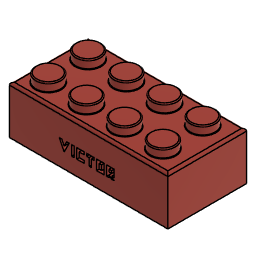
Week 2_Task 1_Ohene (Autodesk Fusion 360 design; units mm, degrees)
Autodesk Fusion 360 part; units mm, degrees
sketch "Sketch1" plane through (0, 0, 0) normal (0, 0, 1) x (1, 0, 0) in component "2x8 Block"
  line L0 (0, 0) -> (31.8, 0)
  line L1 (31.8, 0) -> (31.8, 15.8)
  line L2 (31.8, 15.8) -> (0, 15.8)
  line L3 (0, 15.8) -> (0, 0)
  dimension "d1" = 31.8
  dimension "d2" = 15.8
  constraint horizontal L0
  constraint vertical L1
  constraint horizontal L2
  constraint vertical L3
  constraint coincident L0.start L3.end
  measures "d1" distance of L0.start L0.end
  measures "d2" distance of L0.start L2.end
extrude "Extrude1" add sketch "Sketch1" along normal blind 9.6 in component "2x8 Block"
sketch "Sketch2" plane through (0, 0, 9.6) normal (0, 0, 1) x (-1, 0, 0) in component "2x8 Block"
  line L0 (0, -15.8) -> (0, 0)
  line L1 (0, 0) -> (-31.8, 0)
  line L2 (-31.8, 0) -> (-31.8, -15.8)
  line L3 (-31.8, -15.8) -> (0, -15.8)
  circle A0 centre (-3.9, -11.9) radius 2.5
  dimension "d5" = 5
  dimension "d6" = 3.9
  dimension "d7" = 3.9
  measures "d5" diameter of A0
  measures "d6" distance of L3 A0.centre
  measures "d7" distance of L0 A0.centre
extrude "Extrude2" add sketch "Sketch2" along normal blind 1.7 contours A0 in component "2x8 Block"
pattern_linear "R-Pattern1" count 2 spacing 8 along (0, -1, 0) count 4 spacing 7.6667 along (1, 0, 0) of "Extrude2" in component "2x8 Block"
shell "Shell1" thickness 1.49 removed faces 1 at (21.2, 5.2667, 0) in component "2x8 Block"
sketch "Sketch3" plane through (0, 0, 8.11) normal (0, 0, -1) x (1, 0, 0) in component "2x8 Block"
  circle A0 centre (26.9, -3.9) radius 1.01
  circle A1 centre (26.9, -11.9) radius 1.01
  circle A2 centre (19.2333, -3.9) radius 1.01
  circle A3 centre (19.2333, -11.9) radius 1.01
  circle A4 centre (11.5667, -3.9) radius 1.01
  circle A5 centre (11.5667, -11.9) radius 1.01
  circle A6 centre (3.9, -3.9) radius 1.01
  circle A7 centre (3.9, -11.9) radius 1.01
  line L0 (1.49, -1.49) -> (1.49, -14.31)
  line L1 (1.49, -14.31) -> (30.31, -14.31)
  line L2 (30.31, -14.31) -> (30.31, -1.49)
  line L3 (30.31, -1.49) -> (1.49, -1.49)
  line L4 (11.5667, -3.9) -> (3.9, -11.9) construction
  circle A8 centre (7.7333, -7.9) radius 3.15
  circle A9 centre (7.7333, -7.9) radius 2.15
  dimension "d15" = 6.3
  dimension "d16" = -1
  constraint coincident A4.centre L4.start
  constraint coincident A7.centre L4.end
  constraint midpoint L4 A8.centre
  measures "d15" diameter of A8
extrude "Extrude3" add sketch "Sketch3" along normal blind 8.1 contours A8 in component "2x8 Block"
pattern_linear "R-Pattern2" count 3 spacing 8 along (1, 0, 0) of "Extrude3" in component "2x8 Block"
fillet "Fillet1" radius 0.2 8 edges at (6.2308, 12.804, 11.3) (6.2308, 4.804, 11.3) (13.8975, 4.804, 11.3) (13.8975, 12.804, 11.3) (21.5642, 12.804, 11.3) (21.5642, 4.804, 11.3) (29.2308, 4.804, 11.3) (29.2308, 12.804, 11.3) in component "2x8 Block"
fillet "Fillet2" radius 0.1 8 edges at (6.2308, 10.996, 9.6) (13.8975, 10.996, 9.6) (6.2308, 2.996, 9.6) (13.8975, 2.996, 9.6) (21.5642, 2.996, 9.6) (21.5642, 10.996, 9.6) (29.2308, 10.996, 9.6) (29.2308, 2.996, 9.6) in component "2x8 Block"
fillet "Fillet3" radius 0.5 4 edges at (0, 7.9, 9.6) (15.9, 15.8, 9.6) (15.9, 0, 9.6) (31.8, 7.9, 9.6) in component "2x8 Block"
sketch "Sketch4" plane through (0, 0, 0) normal (0, -1, 0) x (1, 0, 0) in component "2x8 Block"
  line L0 (31.8, 9.1) -> (0, 9.1)
  line L1 (0, 9.1) -> (0, 0)
  line L2 (0, 0) -> (31.8, 0)
  line L3 (31.8, 0) -> (31.8, 9.1)
  line L4 (11, 3) -> (10, 5)
  line L5 (10, 5) -> (10.5, 5)
  line L6 (10.5, 5) -> (11, 4)
  line L7 (11, 4) -> (11.5, 5)
  line L8 (11.5, 5) -> (12, 5)
  line L9 (12, 5) -> (11, 3)
  line L10 (12.5, 5) -> (13, 5)
  line L11 (13, 5) -> (13, 3)
  line L12 (13, 3) -> (12.5, 3)
  line L13 (12.5, 3) -> (12.5, 5)
  line L14 (15, 4.5) -> (15, 5)
  line L15 (15, 5) -> (13.5, 5)
  line L16 (13.5, 5) -> (13.5, 3)
  line L17 (13.5, 3) -> (15, 3)
  line L18 (15, 3) -> (15, 3.5)
  line L19 (15, 3.5) -> (14, 3.5)
  line L20 (14, 3.5) -> (14, 4.5)
  line L21 (14, 4.5) -> (15, 4.5)
  line L22 (15.5, 5) -> (15.5, 4.5)
  line L23 (15.5, 4.5) -> (16, 4.5)
  line L24 (16, 4.5) -> (16, 3)
  line L25 (16, 3) -> (16.4466, 3)
  line L26 (16.4466, 3) -> (16.4466, 4.5)
  line L27 (16.4466, 4.5) -> (17, 4.5)
  line L28 (17, 4.5) -> (17, 5)
  line L29 (17, 5) -> (15.5, 5)
  line L30 (17.5, 5) -> (19, 5)
  line L31 (19, 5) -> (19, 3)
  line L32 (19, 3) -> (17.5, 3)
  line L33 (17.5, 3) -> (17.5, 5)
  line L34 (18, 3.5) -> (18.5, 3.5)
  line L35 (18.5, 3.5) -> (18.5, 4.5)
  line L36 (18.5, 4.5) -> (18, 4.5)
  line L37 (18, 4.5) -> (18, 3.5)
  line L38 (19.5, 5) -> (19.5, 3)
  line L39 (19.5, 3) -> (20, 3)
  line L40 (20, 3) -> (20, 3.5)
  line L41 (20, 3.5) -> (20.5, 3)
  line L42 (20.5, 3) -> (21, 3)
  line L43 (21, 3) -> (20.5, 3.5)
  line L44 (20.5, 3.5) -> (21, 3.5)
  line L45 (21, 3.5) -> (21, 5)
  line L46 (21, 5) -> (19.5, 5)
  line L47 (20, 4) -> (20.5, 4)
  line L48 (20.5, 4) -> (20.5, 4.5)
  line L49 (20.5, 4.5) -> (20, 4.5)
  line L50 (20, 4.5) -> (20, 4)
  constraint horizontal L5
  constraint parallel L4 L6
  constraint parallel L5 L8
  constraint parallel L7 L9
  constraint horizontal L10
  constraint vertical L11
  constraint horizontal L12
  constraint vertical L13
  constraint vertical L14
  constraint perpendicular L14 L15
  constraint perpendicular L15 L16
  constraint perpendicular L16 L17
  constraint perpendicular L17 L18
  constraint perpendicular L16 L19
  constraint perpendicular L19 L20
  constraint perpendicular L14 L21
  constraint perpendicular L21 L22
  constraint perpendicular L22 L23
  constraint perpendicular L23 L24
  constraint perpendicular L24 L25
  constraint perpendicular L25 L26
  constraint perpendicular L24 L27
  constraint perpendicular L25 L28
  constraint perpendicular L22 L29
  constraint horizontal L30
  constraint vertical L31
  constraint horizontal L32
  constraint vertical L33
  constraint horizontal L34
  constraint vertical L35
  constraint horizontal L36
  constraint vertical L37
  constraint vertical L38
  constraint perpendicular L38 L39
  constraint perpendicular L39 L40
  constraint perpendicular L40 L42
  constraint parallel L41 L43
  constraint parallel L42 L44
  constraint perpendicular L44 L45
  constraint perpendicular L38 L46
  constraint horizontal L47
  constraint vertical L48
  constraint horizontal L49
  constraint vertical L50
extrude "Extrude4" cut sketch "Sketch4" against normal blind 1 contours L4 L5 L6 L7 L8 L9 | L10 L11 L12 L13 | L14 L15 L16 L17 L18 L19 L20 L21 | L22 L23 L24 L25 L26 L27 L28 L29 | L30 L31 L32 L33 | L38 L39 L40 L41 L42 L43 L44 L45 L46 in component "2x8 Block"
component "2x8 Block" placed x (1, 0, 0) y (0, 1, 0) z (0, 0, 1) at (0, 0, 0)
